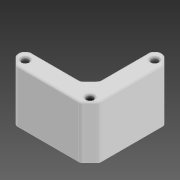
# Autodesk Inventor part: stepper spacer
Saved by Autodesk Inventor 2020 (Build 240168000, 168)
## iProperties
Created: 2020-05-18
Part Number: stepper spacer
Material: Generic
Document SubType Name: Modeling
Designer: stefa
Density: 1 g/cm^3
Appearance: Default
Author: stefa
Autodesk Inventor part; units mm, degrees
ref_plane "YZ Plane" through (0, 0, 0) normal (1, 0, 0) x (0, 1, 0)
ref_plane "XZ Plane" through (0, 0, 0) normal (0, 1, 0) x (-1, 0, 0)
ref_plane "XY Plane" through (0, 0, 0) normal (0, 0, 1) x (1, 0, 0)
sketch "Sketch1" plane through (0, 0, 0) normal (0, 1, 0) x (-1, 0, 0)
  line L0 (0, 0) -> (0, -35.5002)
  line L1 (9, -9) -> (35.5, -9)
  line L2 (35.5002, 0) -> (0, 0)
  circle A0 centre (4.5, -4.5) radius 1.6
  circle A1 centre (35.5, -4.5) radius 1.6
  circle A2 centre (4.5, -35.5) radius 1.6
  line L3 (9, -35.5) -> (9, -9)
  line L4 (31, -9) -> (40, -9)
  line L5 (40, -9) -> (40, 0)
  line L6 (40, 0) -> (31, 0)
  line L7 (31, -9) -> (40, 0) construction
  line L8 (40, -9) -> (31, 0) construction
  line L9 (0, -31) -> (0, -40)
  line L10 (0, -40) -> (9, -40)
  line L11 (9, -40) -> (9, -31)
  line L12 (9, -31) -> (0, -40) construction
  line L13 (0, -31) -> (9, -40) construction
  arc A3 (35.4998, 0) -> (35.4998, 0) centre (35.5, -4.5) ccw
  point P0 (0, 0)
  point P1 (0, -9)
  dimension "d8" = 3.2
  dimension "d21" = 4.5
  dimension "d22" = 31
  dimension "d23" = 31
  dimension "d38" = 4.5
  constraints: 29 end point, 4 centre point, 4 midpoint, 4 point on line, 3 parallel, 3 point on circle, 2 coincident, 2 equal radius, 2 perpendicular, 2 vertical, 1 horizontal, 1 horizontal alignment, 1 vertical alignment
  measures "d8" diameter of A0
  measures "d21" distance from line of L0 A0.centre
  measures "d22" distance of A2.centre A0.centre
  measures "d23" distance of A1.centre A0.centre
  measures "d38" distance from line of L2 A0.centre
extrude "Extrusion1" add sketch "Sketch1" along normal blind 25
chamfer "Chamfer2" distance 2 angle 45 2 edges at (-40, 12.5, -9) (-9, 12.5, -40)
chamfer "Chamfer3" distance 4.5 angle 45 4 edges at (-40, 12.5, 0) (0, 12.5, 0) (0, 12.5, -40) (-9, 12.5, -9)
fillet "Fillet4" radius 2 12 edges at (-40, 12.5, -7) (-35.5, 12.5, 0) (-40, 12.5, -4.5) (-38, 12.5, -9) (-9, 12.5, -38) (-7, 12.5, -40) (-4.5, 12.5, -40) (0, 12.5, -35.5) (0, 12.5, -4.5) (-4.5, 12.5, 0) (-13.5, 12.5, -9) (-9, 12.5, -13.5)
fillet "Fillet5" radius 0.5 23 edges at (-4.5631, 25, -0.1522) (-2.25, 25, -2.25) (-0.1522, 25, -4.5631) (0, 25, -20) (-0.1522, 25, -35.4369) (-2.25, 25, -37.75) (-4.5631, 25, -39.8478) (-5.75, 25, -40) (-6.9369, 25, -39.8478) (-8, 25, -39) (-8.8478, 25, -37.9369) (-9, 25, -24.9142) (-9, 25, -36.3358) (-24.9142, 25, -9) (-36.3358, 25, -9) (-37.9369, 25, -8.8478) (-39, 25, -8) (-39.8478, 25, -6.9369) (-40, 25, -5.75) (-39.8478, 25, -4.5631) (-37.75, 25, -2.25) (-35.4369, 25, -0.1522) (-20, 25, 0)
chamfer "Chamfer4" distance 0.5 angle 45 3 edges at (-33.9, 25, -4.5) (-2.9, 25, -4.5) (-2.9, 25, -35.5)
body "Solid1"
